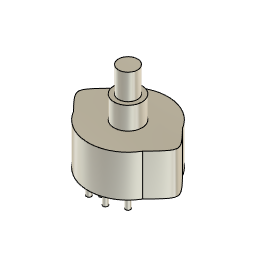
Rotery switch v2 (Autodesk Fusion 360 design; units mm, degrees)
Autodesk Fusion 360 part; units mm, degrees
sketch "Sketch1" plane through (0, 0, 0) normal (0, 0, 1) x (1, 0, 0)
  circle A0 centre (0, 0) radius 12.5
  line L0 (0, 0) -> (12.5, 0) construction
  line L1 (0, 0) -> (12.5059, 0) construction
  spline S0 degree 2 poles (10.8227, -6.2546) (17, 0) (10.8253, 6.25) knots 0 0 0 1.56255 1.56255 1.56255 weights 1 3.141727 1
  line L2 (0, 0) -> (12.5, 0) construction
  line L3 (0, 0) -> (12.5, 0) construction
  spline S1 degree 2 poles (-10.8253, -6.25) (-17, 0) (-10.8253, 6.25) knots 0 0 0 1.561767 1.561767 1.561767 weights 1 3.134953 1
  dimension "d1" = 25
  constraint coincident A0.centre L0.start
  constraint horizontal L0
  constraint horizontal L1
  constraint horizontal L2
  constraint horizontal L3
  constraint coincident A0 S0.start
  measures "d1" diameter of A0
extrude "Extrude1" add sketch "Sketch1" along normal blind 13
sketch "Sketch2" plane through (0, 0, 13) normal (0, 0, 1) x (-1, 0, 0)
  spline S0 degree 2 poles (-10.8227, 6.2546) (-17, 0) (-10.8253, -6.25) knots 0 0 0 1.56255 1.56255 1.56255 weights 1 3.141727 1
  arc A0 (-10.8253, -6.25) -> (10.8253, -6.25) centre (0, 0) ccw
  spline S1 degree 2 poles (10.8253, -6.25) (17, 0) (10.8253, 6.25) knots -1.561767 -1.561767 -1.561767 0 0 0 weights 1 3.134953 1
  arc A1 (10.8253, 6.25) -> (-10.8227, 6.2546) centre (0, 0) ccw
  circle A2 centre (0, 0) radius 4.4
  dimension "d11" = 8.8
  constraint coincident A0.centre A1.centre
  measures "d11" diameter of A2
extrude "Extrude2" add sketch "Sketch2" along normal blind 7 contours A2
sketch "Sketch3" plane through (0, 0, 20) normal (0, 0, 1) x (-1, 0, 0)
  circle A0 centre (0, 0) radius 4.4
cylinder "CylinderPrimitive1" add diameter 6 height 8 placed x (1, 0, 0) y (0, 1, 0) z (0, 0, 1) at (0, 0, 20)
sketch "Sketch4" plane through (0, 0, 20) normal (0, 0, 1) x (-1, 0, 0)
sketch "Sketch5" plane through (0, 0, 0) normal (0, 0, -1) x (1, 0, 0)
  spline S0 degree 2 poles (10.8227, 6.2546) (17, 0) (10.8253, -6.25) knots 0 0 0 1.56255 1.56255 1.56255 weights 1 3.141727 1
  arc A0 (10.8227, 6.2546) -> (-10.8253, 6.25) centre (0, 0) ccw
  spline S1 degree 2 poles (-10.8253, 6.25) (-17, 0) (-10.8253, -6.25) knots 0 0 0 1.561767 1.561767 1.561767 weights 1 3.134953 1
  arc A1 (-10.8253, -6.25) -> (10.8253, -6.25) centre (0, 0) ccw
  line L0 (0, 0) -> (10, 0) construction
  line L1 (0, 0) -> (10, 0) construction
  circle A2 centre (-9.6593, -2.5882) radius 0.75
  circle A3 centre (-9.6593, 2.5882) radius 0.75
  circle A4 centre (-7.0711, 7.0711) radius 0.75
  circle A5 centre (-2.5882, 9.6593) radius 0.75
  circle A6 centre (2.5882, 9.6593) radius 0.75
  circle A7 centre (7.0711, 7.0711) radius 0.75
  dimension "d19" = 1.5
  dimension "d21" = -150
  constraint horizontal L0
  constraint coincident A0.centre A1.centre
  constraint horizontal L1
  measures "d19" diameter of A2
extrude "Extrude3" add sketch "Sketch5" along normal blind 4 contours A2 | A3 | A4 | A5 | A6 | A7
sketch "Sketch6" plane through (0, 0, 0) normal (0, 0, -1) x (1, 0, 0)
  circle A0 centre (7.0711, 7.0711) radius 0.75
  circle A1 centre (-9.6593, 2.5882) radius 0.75
  circle A2 centre (-7.0711, 7.0711) radius 0.75
  circle A3 centre (2.5882, 9.6593) radius 0.75
  circle A4 centre (-9.6593, -2.5882) radius 0.75
  circle A5 centre (-2.5882, 9.6593) radius 0.75
  spline S0 degree 2 poles (10.8227, 6.2546) (17, 0) (10.8253, -6.25) knots 0 0 0 1.56255 1.56255 1.56255 weights 1 3.141727 1
  arc A6 (10.8227, 6.2546) -> (-10.8253, 6.25) centre (0, 0) ccw
  spline S1 degree 2 poles (-10.8253, 6.25) (-17, 0) (-10.8253, -6.25) knots 0 0 0 1.561767 1.561767 1.561767 weights 1 3.134953 1
  arc A7 (-10.8253, -6.25) -> (10.8253, -6.25) centre (0, 0) ccw
  line L0 (0, 0) -> (6, 0) construction
  circle A8 centre (-3, 5.1962) radius 0.75
  dimension "d26" = 1.5
  constraint horizontal L0
  constraint coincident A6.centre A7.centre
  measures "d26" diameter of A8
extrude "Extrude4" add sketch "Sketch6" along normal blind 6.5 contours A8
